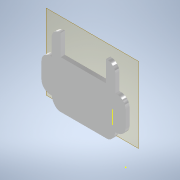
# Autodesk Inventor part: bottom-bracket
Saved by Autodesk Inventor 2020 (Build 240168000, 168)
## iProperties
Created: 2019-11-08
Part Number: bottom-bracket
Material: Aluminum 6061
Document SubType Name: Modeling
Designer: Hymowitz
Density: 2.7 g/cm^3
Sheet Metal Width: 0.000 in
Sheet Metal Length: 0.000 in
Sheet Metal Area: 0.000 in^2
Appearance: Aluminum - Flat
Author: Hymowitz
Autodesk Inventor part; units mm, degrees
ref_plane "YZ Plane" through (0, 0, 0) normal (1, 0, 0) x (0, 1, 0)
ref_plane "XZ Plane" through (0, 0, 0) normal (0, 1, 0) x (-1, 0, 0)
ref_plane "XY Plane" through (0, 0, 0) normal (0, 0, 1) x (1, 0, 0)
ref_plane "Work Plane1" through (3.6062, 5.0251, 0) normal (0, 0, 1) x (1, 0, 0)
sketch "Sketch1" plane through (3.6062, 5.0251, 0) normal (0, 0, 1) x (1, 0, 0)
  line L0 (-59.3453, 14.0249) -> (-60.5022, 14.0249)
  ellipse E0 centre (-52.8822, 15.9436) end of major axis (-52.8822, 6.6041) minor radius 6.604 (-59.3453, 14.0249) -> (-52.8822, 6.6041) ccw
  line L1 (-52.8822, 6.6041) -> (-17.8302, 6.6041)
  ellipse E1 centre (-17.8302, 15.9436) end of major axis (-17.8302, 25.2831) minor radius 6.604 (-17.8302, 6.6041) -> (-11.367, 14.0249) ccw
  line L2 (-10.2102, 14.0249) -> (-11.367, 14.0249)
  arc A0 (-10.2102, 14.0249) -> (-3.6062, 20.6289) centre (-10.2102, 20.6289) ccw
  line L3 (-3.6062, 20.6289) -> (-3.6062, 32.8209)
  arc A1 (-3.6062, 32.8209) -> (-10.2102, 39.4249) centre (-10.2102, 32.8209) ccw
  line L4 (-11.2262, 39.4249) -> (-10.2102, 39.4249)
  line L5 (-11.2262, 51.8709) -> (-11.2262, 39.4249)
  arc A2 (-11.2262, 51.8709) -> (-17.8302, 58.4749) centre (-17.8302, 51.8709) ccw
  line L6 (-17.8302, 58.4749) -> (-52.8822, 58.4749)
  arc A3 (-52.8822, 58.4749) -> (-59.4862, 51.8709) centre (-52.8822, 51.8709) ccw
  line L7 (-59.4862, 39.4249) -> (-59.4862, 51.8709)
  line L8 (-60.5022, 39.4249) -> (-59.4862, 39.4249)
  arc A4 (-60.5022, 39.4249) -> (-67.1062, 32.8209) centre (-60.5022, 32.8209) ccw
  line L9 (-67.1062, 20.6289) -> (-67.1062, 32.8209)
  arc A5 (-67.1062, 20.6289) -> (-60.5022, 14.0249) centre (-60.5022, 20.6289) ccw
  line L10 (-52.8822, 6.6041) -> (-17.8302, 6.6041)
  point P0 (-3.6062, -5.0251)
extrude "Plate1" add sketch "Sketch1" along normal blind 3.048
sketch "Sketch2" plane through (3.6062, 5.0251, 3.048) normal (0, 0, 1) x (1, 0, 0)
  line L0 (-19.2272, 69.2699) -> (-19.2272, 51.2359) projected
  line L1 (-42.2142, 43.5397) -> (-28.4982, 43.5397) projected
  line L2 (-51.4852, 51.2359) -> (-51.4852, 69.2699) projected
  line L3 (-19.2272, 58.5208) -> (-19.2272, 43.5397)
  line L4 (-19.2272, 43.5397) -> (-51.4852, 43.5397)
  line L5 (-51.4852, 43.5397) -> (-51.4852, 64.3147)
  line L6 (-52.4852, 58.4749) -> (-52.4852, 42.5397)
  line L7 (-52.4852, 42.5397) -> (-18.2272, 42.5397)
  line L8 (-18.2272, 42.5397) -> (-18.2272, 58.5208)
  line L9 (-52.8822, 58.4749) -> (-17.8302, 58.4749) projected
  point P0 (0, 0)
  point P1 (-18.2272, 58.4749)
  dimension "d2" = 1
  constraints: 12 end point, 3 point on line, 1 vertical, 2 other
  measures "d2" distance between parallel lines of L4 L7
extrude "Extrusion2" cut sketch "Sketch2" against normal through all
sketch "Sketch4" plane through (3.6062, 5.0251, 3.048) normal (0, 0, 1) x (1, 0, 0)
  line L0 (-12.8862, 21.4549) -> (-12.8862, 17.4549) projected
  line L1 (-9.0098, 35.2125) -> (-13.2052, 35.2125)
  line L2 (-13.2052, 35.2125) -> (-13.2052, 18.2304)
  line L3 (-13.2052, 18.2304) -> (-9.0098, 18.2304)
  line L4 (-9.0098, 18.2304) -> (-9.0098, 35.2125)
  line L5 (-9.0098, 35.2125) -> (-13.2052, 18.2304) construction
  line L6 (-13.2052, 35.2125) -> (-9.0098, 18.2304) construction
  line L7 (-12.8862, 21.4549) -> (-12.8862, 17.4549) projected
  point P0 (-3.6062, -5.0251)
  point P1 (-11.1075, 26.7215)
  point P2 (-11.1075, 26.7215)
  dimension "d18" = 4.1954
  constraints: 12 end point, 3 midpoint, 2 parallel, 1 horizontal, 1 perpendicular, 1 other
  measures "d18" distance between parallel lines of L4 L2
extrude "Extrusion3" cut sketch "Sketch4" against normal blind 2
equation "\"d5\" = Thickness"
equation "\"BendRadius\" = Thickness"
equation "\"BendReliefWidth\" = Thickness"
equation "\"BendReliefDepth\" = 0.5 * Thickness"
equation "\"CornerReliefSize\" = 4 * Thickness"
equation "\"MinimumRemnant\" = 2 * Thickness"
equation "\"TransitionRadius\" = BendRadius"
equation "\"JacobiRadiusSize\" = Thickness"
equation "\"GapSize\" = Thickness"
equation "\"Thickness\" = 3.048"
body "Solid1"
